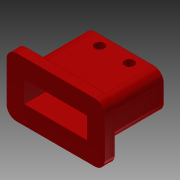
# Autodesk Inventor part: E-Stop_Fixture_Tall
Saved by Autodesk Inventor 2015 (Build 190159000, 159)
## iProperties
Created: 2015-01-06
Part Number: E-Stop_Fixture_Tall
Material: Generic
Document SubType Name: Modeling
Designer: Drew
Density: 1 g/cm^3
Appearance: Smooth - Red
Author: Drew
Autodesk Inventor part; units mm, degrees
ref_plane "YZ Plane" through (0, 0, 0) normal (1, 0, 0) x (0, 1, 0)
ref_plane "XZ Plane" through (0, 0, 0) normal (0, 1, 0) x (-1, 0, 0)
ref_plane "XY Plane" through (0, 0, 0) normal (0, 0, 1) x (1, 0, 0)
sketch "Sketch1" plane through (0, 0, 0) normal (0, 0, 1) x (1, 0, 0)
  line L0 (12.7, -6.0198) -> (-12.7, -6.0198)
  line L1 (-12.7, -6.0198) -> (-12.7, 6.0198)
  line L2 (-12.7, 6.0198) -> (12.7, 6.0198)
  line L3 (12.7, 6.0198) -> (12.7, -6.0198)
  line L4 (12.7, -6.0198) -> (-12.7, 6.0198) construction
  line L5 (-12.7, -6.0198) -> (12.7, 6.0198) construction
  point P0 (0, 0)
  dimension "d0" = 25.4
  dimension "d1" = 12.0396
  constraints: 12 end point, 2 midpoint, 2 parallel, 1 horizontal, 1 perpendicular
  measures "d0" distance of L1.end L2.end
  measures "d1" distance of L0.end L1.end
extrude "Extrusion1" add sketch "Sketch1" along normal blind 19.05
shell "Shell1" thickness 2.54 removed faces 2 at (4.2333, -2.0066, 0) at (4.2333, -2.0066, 19.05)
sketch "Sketch2" plane through (-12.7, 6.0198, 0) normal (0, 1, 0) x (1, 0, 0)
  line L0 (-2.1226, -3.175) -> (30.0619, -3.175)
  line L1 (0, 0) -> (25.4, 0) projected
  circle A0 centre (7.874, -3.175) radius 1.524
  circle A1 centre (17.526, -3.175) radius 1.524
  line L2 (12.7, 1.1779) -> (12.7, -16.2415)
  point P0 (12.7, 0)
  point P1 (12.7, 0)
  dimension "d23" = 3.175
  dimension "d24" = 3.048
  dimension "d25" = 9.652
  constraints: 4 end point, 3 point on line, 2 centre point, 1 horizontal, 1 midpoint, 1 parallel, 1 vertical, 1 other
  measures "d23" distance between parallel lines of L0 L1
  measures "d24" diameter of A0
  measures "d25" distance of A1.centre A0.centre
extrude "Extrusion2" cut sketch "Sketch2" against normal through all
sketch "Sketch3" plane through (0, 0, 19.05) normal (0, 0, 1) x (1, 0, 0)
  line L0 (-10.16, 3.4798) -> (10.16, 3.4798)
  line L1 (10.16, 3.4798) -> (10.16, -3.4798)
  line L2 (10.16, -3.4798) -> (-10.16, -3.4798)
  line L3 (-10.16, -3.4798) -> (-10.16, 3.4798)
  line L4 (-10.16, 3.4798) -> (10.16, -3.4798) construction
  line L5 (10.16, 3.4798) -> (-10.16, -3.4798) construction
  line L6 (-12.7, 9.525) -> (12.7, 9.525)
  line L7 (15.875, 6.35) -> (15.875, -6.35)
  line L8 (12.7, -9.525) -> (-12.7, -9.525)
  line L9 (-15.875, -6.35) -> (-15.875, 6.35)
  line L10 (-15.875, 9.525) -> (15.875, -9.525) construction
  line L11 (15.875, 9.525) -> (-15.875, -9.525) construction
  arc A0 (12.7, -9.525) -> (15.875, -6.35) centre (12.7, -6.35) ccw
  arc A1 (15.875, 6.35) -> (12.7, 9.525) centre (12.7, 6.35) ccw
  arc A2 (-12.7, 9.525) -> (-15.875, 6.35) centre (-12.7, 6.35) ccw
  arc A3 (-15.875, -6.35) -> (-12.7, -9.525) centre (-12.7, -6.35) ccw
  point P0 (0, 0)
  dimension "d28" = 19.05
  dimension "d29" = 31.75
  dimension "d30" = 3.175
  constraints: 24 end point, 8 point on circle, 8 point on line, 8 tangent, 4 centre point, 4 midpoint, 4 parallel, 3 equal radius, 2 horizontal, 2 perpendicular
  measures "d28" distance of L11.start L10.end
  measures "d29" distance of L10.end L11.end
  measures "d30" radius of A0
extrude "Extrusion3" add sketch "Sketch3" along normal blind 3.175
fillet "Fillet1" radius 3.175 4 edges at (12.7, 6.0198, 9.525) (12.7, -6.0198, 9.525) (-12.7, 6.0198, 9.525) (-12.7, -6.0198, 9.525)
body "Solid1"
